Autodesk Fusion 360 part; units mm, degrees
note: some values were not read from the file. Chosen so that the rebuilt part matches the saved one: that a step has no effect.
(part 4 of 7)
  spline S1007 degree 3 poles (-9.5703, 47.6755) (-12.0382, 47.6755) (-14.506, 47.6755) (-17.0486, 47.6755) knots 0 0 0 0 1 1 1 1
  spline S1008 degree 3 poles (-17.0486, 47.6755) (-17.2132, 47.1819) (-17.3777, 46.6884) (-17.5472, 46.1798) knots 0 0 0 0 1 1 1 1
  spline S1009 degree 3 poles (-17.5472, 46.1798) (-17.5472, 46.8379) (-17.5472, 47.496) (-17.5472, 48.1741) knots 0 0 0 0 1 1 1 1
  spline S1010 degree 3 poles (-17.5472, 48.1741) (-16.019, 48.9382) (-14.4225, 48.7239) (-12.7486, 48.7038) knots 0 0 0 0 1 1 1 1
  spline S1011 degree 3 poles (-38.4866, -11.6527) (-38.4866, -12.1462) (-38.4866, -12.6398) (-38.4866, -13.1483) knots 0 0 0 0 1 1 1 1
  spline S1012 degree 3 poles (-38.4866, -13.1483) (-41.777, -13.1483) (-45.0675, -13.1483) (-48.4577, -13.1483) knots 0 0 0 0 1 1 1 1
  spline S1013 degree 3 poles (-48.4577, -13.1483) (-48.4577, -12.8193) (-48.4577, -12.4902) (-48.4577, -12.1512) knots 0 0 0 0 1 1 1 1
  spline S1014 degree 3 poles (-48.4577, -12.1512) (-45.1391, -11.5338) (-41.8532, -11.6071) (-38.4866, -11.6527) knots 0 0 0 0 1 1 1 1
  spline S1015 degree 3 poles (38.2911, 14.2723) (38.1265, 12.9561) (37.962, 11.6399) (37.7925, 10.2838) knots 0 0 0 0 1 1 1 1
  spline S1016 degree 3 poles (37.7925, 10.2838) (37.628, 10.7774) (37.4635, 11.271) (37.294, 11.7795) knots 0 0 0 0 1 1 1 1
  spline S1017 degree 3 poles (37.294, 11.7795) (36.0132, 12.4199) (34.918, 12.4424) (33.4925, 12.5585) knots 0 0 0 0 1 1 1 1
  spline S1018 degree 3 poles (33.4925, 12.5585) (32.9925, 12.6002) (32.4925, 12.642) (31.9773, 12.6851) knots 0 0 0 0 1 1 1 1
  spline S1019 degree 3 poles (31.9773, 12.6851) (31.593, 12.7153) (31.2087, 12.7455) (30.8127, 12.7766) knots 0 0 0 0 1 1 1 1
  spline S1020 degree 3 poles (30.8127, 12.7766) (30.8127, 12.9411) (30.8127, 13.1056) (30.8127, 13.2751) knots 0 0 0 0 1 1 1 1
  spline S1021 degree 3 poles (30.8127, 13.2751) (33.3428, 13.9049) (35.6627, 14.407) (38.2911, 14.2723) knots 0 0 0 0 1 1 1 1
  spline S1022 degree 3 poles (-34.9967, -11.6527) (-34.8321, -11.9817) (-34.6676, -12.3107) (-34.4981, -12.6498) knots 0 0 0 0 1 1 1 1
  spline S1023 degree 3 poles (-34.4981, -12.6498) (-33.84, -12.4852) (-33.1819, -12.3207) (-32.5039, -12.1512) knots 0 0 0 0 1 1 1 1
  spline S1024 degree 3 poles (-32.5039, -12.1512) (-32.5039, -12.3157) (-32.5039, -12.4803) (-32.5039, -12.6498) knots 0 0 0 0 1 1 1 1
  spline S1025 degree 3 poles (-32.5039, -12.6498) (-30.6941, -12.8143) (-28.8844, -12.9788) (-27.0198, -13.1483) knots 0 0 0 0 1 1 1 1
  spline S1026 degree 3 poles (-27.0198, -13.1483) (-26.8552, -12.8193) (-26.6907, -12.4902) (-26.5212, -12.1512) knots 0 0 0 0 1 1 1 1
  spline S1027 degree 3 poles (-26.5212, -12.1512) (-25.4929, -11.8396) (-25.4929, -11.8396) (-24.527, -11.6527) knots 0 0 0 0 1 1 1 1
  spline S1028 degree 3 poles (-24.527, -11.6527) (-24.527, -12.3107) (-24.527, -12.9688) (-24.527, -13.6469) knots 0 0 0 0 1 1 1 1
  spline S1029 degree 3 poles (-24.527, -13.6469) (-27.8175, -13.6469) (-31.1079, -13.6469) (-34.4981, -13.6469) knots 0 0 0 0 1 1 1 1
  spline S1030 degree 3 poles (-34.4981, -13.6469) (-34.6626, -12.9888) (-34.8272, -12.3307) (-34.9967, -11.6527) knots 0 0 0 0 1 1 1 1
  spline S1031 degree 3 poles (-8.0746, 35.2116) (-7.9101, 35.2116) (-7.7456, 35.2116) (-7.5761, 35.2116) knots 0 0 0 0 1 1 1 1
  spline S1032 degree 3 poles (-7.5761, 35.2116) (-7.5761, 34.389) (-7.5761, 33.5664) (-7.5761, 32.7188) knots 0 0 0 0 1 1 1 1
  spline S1033 degree 3 poles (-7.5761, 32.7188) (-6.918, 32.7188) (-6.2599, 32.7188) (-5.5819, 32.7188) knots 0 0 0 0 1 1 1 1
  spline S1034 degree 3 poles (-5.5819, 32.7188) (-5.9109, 31.8962) (-6.24, 31.0736) (-6.579, 30.2261) knots 0 0 0 0 1 1 1 1
  spline S1035 degree 3 poles (-6.579, 30.2261) (-7.2371, 30.7196) (-7.8952, 31.2132) (-8.5732, 31.7217) knots 0 0 0 0 1 1 1 1
  spline S1036 degree 3 poles (-8.5732, 31.7217) (-8.7377, 31.3927) (-8.9022, 31.0636) (-9.0717, 30.7246) knots 0 0 0 0 1 1 1 1
  spline S1037 degree 3 poles (-9.0717, 30.7246) (-10.0589, 30.231) (-10.0589, 30.231) (-11.066, 29.7275) knots 0 0 0 0 1 1 1 1
  spline S1038 degree 3 poles (-11.066, 29.7275) (-10.0788, 31.5373) (-9.0917, 33.347) (-8.0746, 35.2116) knots 0 0 0 0 1 1 1 1
  spline S1039 degree 3 poles (4.8878, -4.6729) (5.6867, -7.0587) (4.9289, -8.9438) (3.8907, -11.1541) knots 0 0 0 0 1 1 1 1
  spline S1040 degree 3 poles (3.8907, -11.1541) (2.8001, -12.1824) (2.8001, -12.1824) (1.8965, -12.6498) knots 0 0 0 0 1 1 1 1
  spline S1041 degree 3 poles (1.8965, -12.6498) (2.7191, -12.8143) (3.5417, -12.9788) (4.3893, -13.1483) knots 0 0 0 0 1 1 1 1
  spline S1042 degree 3 poles (4.3893, -13.1483) (4.3893, -13.3128) (4.3893, -13.4774) (4.3893, -13.6469) knots 0 0 0 0 1 1 1 1
  spline S1043 degree 3 poles (4.3893, -13.6469) (3.2376, -13.6469) (2.0859, -13.6469) (0.8994, -13.6469) knots 0 0 0 0 1 1 1 1
  spline S1044 degree 3 poles (0.8994, -13.6469) (0.8994, -12.9888) (0.8994, -12.3307) (0.8994, -11.6527) knots 0 0 0 0 1 1 1 1
  spline S1045 degree 3 poles (0.8994, -11.6527) (1.2798, -11.2928) (1.6603, -10.9329) (2.0523, -10.5621) knots 0 0 0 0 1 1 1 1
  spline S1046 degree 3 poles (2.0523, -10.5621) (3.7647, -8.77) (4.2569, -7.0271) (4.8878, -4.6729) knots 0 0 0 0 1 1 1 1
  spline S1047 degree 3 poles (-23.0313, 13.7737) (-21.4733, 13.0882) (-21.4733, 13.0882) (-20.5385, 12.278) knots 0 0 0 0 1 1 1 1
  spline S1048 degree 3 poles (-20.5385, 12.278) (-20.5385, 11.949) (-20.5385, 11.6199) (-20.5385, 11.2809) knots 0 0 0 0 1 1 1 1
  spline S1049 degree 3 poles (-20.5385, 11.2809) (-21.0321, 11.1164) (-21.5257, 10.9519) (-22.0342, 10.7824) knots 0 0 0 0 1 1 1 1
  spline S1050 degree 3 poles (-22.0342, 10.7824) (-22.0342, 11.1114) (-22.0342, 11.4405) (-22.0342, 11.7795) knots 0 0 0 0 1 1 1 1
  spline S1051 degree 3 poles (-22.0342, 11.7795) (-22.3633, 11.7795) (-22.6923, 11.7795) (-23.0313, 11.7795) knots 0 0 0 0 1 1 1 1
  spline S1052 degree 3 poles (-23.0313, 11.7795) (-23.0313, 12.1085) (-23.0313, 12.4376) (-23.0313, 12.7766) knots 0 0 0 0 1 1 1 1
  spline S1053 degree 3 poles (-23.0313, 12.7766) (-25.1701, 12.7766) (-27.3089, 12.7766) (-29.5125, 12.7766) knots 0 0 0 0 1 1 1 1
  spline S1054 degree 3 poles (-29.5125, 12.7766) (-27.3952, 14.1881) (-25.5172, 14.0389) (-23.0313, 13.7737) knots 0 0 0 0 1 1 1 1
  spline S1055 degree 3 poles (-67.9014, 21.7506) (-68.5578, 18.9278) (-69.5994, 17.8889) (-71.8898, 16.2665) knots 0 0 0 0 1 1 1 1
  spline S1056 degree 3 poles (-71.8898, 16.2665) (-72.2189, 16.2665) (-72.5479, 16.2665) (-72.8869, 16.2665) knots 0 0 0 0 1 1 1 1
  spline S1057 degree 3 poles (-72.8869, 16.2665) (-72.2127, 17.7316) (-71.4414, 18.905) (-70.3941, 20.1303) knots 0 0 0 0 1 1 1 1
  spline S1058 degree 3 poles (-70.3941, 20.1303) (-70.1371, 20.4362) (-69.88, 20.7421) (-69.6151, 21.0573) knots 0 0 0 0 1 1 1 1
  spline S1059 degree 3 poles (-69.6151, 21.0573) (-68.8985, 21.7506) (-68.8985, 21.7506) (-67.9014, 21.7506) knots 0 0 0 0 1 1 1 1
  spline S1060 degree 3 poles (23.8329, 34.2145) (24.3315, 32.7188) (24.3315, 32.7188) (24.3315, 31.7217) knots 0 0 0 0 1 1 1 1
  spline S1061 degree 3 poles (24.3315, 31.7217) (24.6605, 31.3927) (24.9896, 31.0636) (25.3286, 30.7246) knots 0 0 0 0 1 1 1 1
  spline S1062 degree 3 poles (25.3286, 30.7246) (23.5167, 29.565) (21.9529, 29.6464) (19.8445, 29.7275) knots 0 0 0 0 1 1 1 1
  spline S1063 degree 3 poles (19.8445, 29.7275) (19.68, 30.0565) (19.5155, 30.3856) (19.3459, 30.7246) knots 0 0 0 0 1 1 1 1
  spline S1064 degree 3 poles (19.3459, 30.7246) (20.1686, 30.7246) (20.9912, 30.7246) (21.8387, 30.7246) knots 0 0 0 0 1 1 1 1
  spline S1065 degree 3 poles (21.8387, 30.7246) (21.8387, 31.0537) (21.8387, 31.3827) (21.8387, 31.7217) knots 0 0 0 0 1 1 1 1
  spline S1066 degree 3 poles (21.8387, 31.7217) (22.1678, 31.7217) (22.4968, 31.7217) (22.8358, 31.7217) knots 0 0 0 0 1 1 1 1
  spline S1067 degree 3 poles (22.8358, 31.7217) (22.9078, 32.0405) (22.9798, 32.3592) (23.054, 32.6877) knots 0 0 0 0 1 1 1 1
  spline S1068 degree 3 poles (23.054, 32.6877) (23.3344, 33.7159) (23.3344, 33.7159) (23.8329, 34.2145) knots 0 0 0 0 1 1 1 1
  spline S1069 degree 3 poles (-56.9331, 25.2405) (-54.7943, 25.076) (-52.6555, 24.9114) (-50.4519, 24.7419) knots 0 0 0 0 1 1 1 1
  spline S1070 degree 3 poles (-50.4519, 24.7419) (-50.4519, 23.9193) (-50.4519, 23.0967) (-50.4519, 22.2492) knots 0 0 0 0 1 1 1 1
  spline S1071 degree 3 poles (-50.4519, 22.2492) (-50.727, 22.4073) (-51.002, 22.5653) (-51.2854, 22.7282) knots 0 0 0 0 1 1 1 1
  spline S1072 degree 3 poles (-51.2854, 22.7282) (-52.5881, 23.3096) (-53.6455, 23.4459) (-55.0635, 23.5579) knots 0 0 0 0 1 1 1 1
  spline S1073 degree 3 poles (-55.0635, 23.5579) (-55.5083, 23.5951) (-55.953, 23.6324) (-56.4112, 23.6708) knots 0 0 0 0 1 1 1 1
  spline S1074 degree 3 poles (-56.4112, 23.6708) (-56.9163, 23.7075) (-56.9163, 23.7075) (-57.4317, 23.7448) knots 0 0 0 0 1 1 1 1
  spline S1075 degree 3 poles (-57.4317, 23.7448) (-57.2672, 24.2384) (-57.1026, 24.732) (-56.9331, 25.2405) knots 0 0 0 0 1 1 1 1
  spline S1076 degree 3 poles (-60.9216, -11.6527) (-59.4409, -11.8172) (-57.9602, -11.9817) (-56.4346, -12.1512) knots 0 0 0 0 1 1 1 1
  spline S1077 degree 3 poles (-56.4346, -12.1512) (-58.032, -13.2161) (-58.4268, -13.269) (-60.2575, -13.2457) knots 0 0 0 0 1 1 1 1
  spline S1078 degree 3 poles (-60.2575, -13.2457) (-60.7025, -13.2425) (-61.1476, -13.2393) (-61.6061, -13.236) knots 0 0 0 0 1 1 1 1
  spline S1079 degree 3 poles (-61.6061, -13.236) (-62.3007, -13.2234) (-62.3007, -13.2234) (-63.0093, -13.2106) knots 0 0 0 0 1 1 1 1
  spline S1080 degree 3 poles (-63.0093, -13.2106) (-63.4781, -13.2061) (-63.9469, -13.2016) (-64.43, -13.197) knots 0 0 0 0 1 1 1 1
  spline S1081 degree 3 poles (-64.43, -13.197) (-65.5872, -13.1853) (-66.7442, -13.1689) (-67.9014, -13.1483) knots 0 0 0 0 1 1 1 1
  spline S1082 degree 3 poles (-67.9014, -13.1483) (-67.9014, -12.9838) (-67.9014, -12.8193) (-67.9014, -12.6498) knots 0 0 0 0 1 1 1 1
  spline S1083 degree 3 poles (-67.9014, -12.6498) (-65.598, -12.6498) (-63.2947, -12.6498) (-60.9216, -12.6498) knots 0 0 0 0 1 1 1 1
  spline S1084 degree 3 poles (-60.9216, -12.6498) (-60.9216, -12.3207) (-60.9216, -11.9917) (-60.9216, -11.6527) knots 0 0 0 0 1 1 1 1
  spline S1085 degree 3 poles (-12.5616, -1.6815) (-12.2326, -1.6815) (-11.9035, -1.6815) (-11.5645, -1.6815) knots 0 0 0 0 1 1 1 1
  spline S1086 degree 3 poles (-11.5645, -1.6815) (-11.6352, -2.5542) (-11.7084, -3.4266) (-11.7826, -4.299) knots 0 0 0 0 1 1 1 1
  spline S1087 degree 3 poles (-11.7826, -4.299) (-11.8231, -4.7848) (-11.8636, -5.2707) (-11.9053, -5.7713) knots 0 0 0 0 1 1 1 1
  spline S1088 degree 3 poles (-11.9053, -5.7713) (-12.0385, -6.9486) (-12.2394, -8.0227) (-12.5616, -9.1599) knots 0 0 0 0 1 1 1 1
  spline S1089 degree 3 poles (-12.5616, -9.1599) (-12.5616, -8.8308) (-12.5616, -8.5018) (-12.5616, -8.1628) knots 0 0 0 0 1 1 1 1
  spline S1090 degree 3 poles (-12.5616, -8.1628) (-12.8907, -8.1628) (-13.2197, -8.1628) (-13.5588, -8.1628) knots 0 0 0 0 1 1 1 1
  spline S1091 degree 3 poles (-13.5588, -8.1628) (-14.1196, -5.2961) (-14.1196, -5.2961) (-13.5588, -4.1743) knots 0 0 0 0 1 1 1 1
  spline S1092 degree 3 poles (-13.5588, -4.1743) (-13.2297, -4.1743) (-12.9007, -4.1743) (-12.5616, -4.1743) knots 0 0 0 0 1 1 1 1
  spline S1093 degree 3 poles (-12.5616, -4.1743) (-12.5616, -3.3517) (-12.5616, -2.5291) (-12.5616, -1.6815) knots 0 0 0 0 1 1 1 1
  spline S1094 degree 3 poles (-40.9793, 6.2954) (-40.8148, 6.2954) (-40.6503, 6.2954) (-40.4808, 6.2954) knots 0 0 0 0 1 1 1 1
  spline S1095 degree 3 poles (-40.4808, 6.2954) (-40.402, 2.2758) (-40.402, 2.2758) (-40.9793, 0.3127) knots 0 0 0 0 1 1 1 1
  spline S1096 degree 3 poles (-40.9793, 0.3127) (-41.4729, 0.0659) (-41.4729, 0.0659) (-41.9764, -0.1859) knots 0 0 0 0 1 1 1 1
  spline S1097 degree 3 poles (-41.9764, -0.1859) (-42.5416, -1.1913) (-42.5416, -1.1913) (-42.9736, -2.1801) knots 0 0 0 0 1 1 1 1
  spline S1098 degree 3 poles (-42.9736, -2.1801) (-43.4721, -1.183) (-43.4721, -1.183) (-42.9755, 0.5503) knots 0 0 0 0 1 1 1 1
  spline S1099 degree 3 poles (-42.9755, 0.5503) (-42.7397, 1.241) (-42.5, 1.9304) (-42.2569, 2.6185) knots 0 0 0 0 1 1 1 1
  spline S1100 degree 3 poles (-42.2569, 2.6185) (-42.1357, 2.9707) (-42.0146, 3.3229) (-41.8898, 3.6857) knots 0 0 0 0 1 1 1 1
  spline S1101 degree 3 poles (-41.8898, 3.6857) (-41.5896, 4.5568) (-41.2849, 5.4262) (-40.9793, 6.2954) knots 0 0 0 0 1 1 1 1
  spline S1102 degree 3 poles (41.781, 8.2896) (42.8247, 6.5935) (42.8675, 5.272) (42.7781, 3.304) knots 0 0 0 0 1 1 1 1
  spline S1103 degree 3 poles (42.7781, 3.304) (42.2845, 3.304) (41.7909, 3.304) (41.2824, 3.304) knots 0 0 0 0 1 1 1 1
  spline S1104 degree 3 poles (41.2824, 3.304) (41.2824, 2.4814) (41.2824, 1.6588) (41.2824, 0.8112) knots 0 0 0 0 1 1 1 1
  spline S1105 degree 3 poles (41.2824, 0.8112) (40.9534, 1.1403) (40.6243, 1.4693) (40.2853, 1.8084) knots 0 0 0 0 1 1 1 1
  spline S1106 degree 3 poles (40.2853, 1.8084) (40.4616, 4.1002) (40.9932, 6.1363) (41.781, 8.2896) knots 0 0 0 0 1 1 1 1
  spline S1107 degree 3 poles (-59.9245, 16.765) (-58.4911, 16.8274) (-58.4911, 16.8274) (-56.9331, 16.765) knots 0 0 0 0 1 1 1 1
  spline S1108 degree 3 poles (-56.9331, 16.765) (-55.936, 15.7679) (-55.936, 15.7679) (-55.8737, 14.4592) knots 0 0 0 0 1 1 1 1
  spline S1109 degree 3 poles (-55.8737, 14.4592) (-55.8943, 14.0685) (-55.9148, 13.6777) (-55.936, 13.2751) knots 0 0 0 0 1 1 1 1
  spline S1110 degree 3 poles (-55.936, 13.2751) (-56.4296, 13.2751) (-56.9232, 13.2751) (-57.4317, 13.2751) knots 0 0 0 0 1 1 1 1
  spline S1111 degree 3 poles (-57.4317, 13.2751) (-57.4317, 13.9332) (-57.4317, 14.5913) (-57.4317, 15.2694) knots 0 0 0 0 1 1 1 1
  spline S1112 degree 3 poles (-57.4317, 15.2694) (-58.2543, 15.2694) (-59.0769, 15.2694) (-59.9245, 15.2694) knots 0 0 0 0 1 1 1 1
  spline S1113 degree 3 poles (-59.9245, 15.2694) (-59.9245, 15.7629) (-59.9245, 16.2565) (-59.9245, 16.765) knots 0 0 0 0 1 1 1 1
  spline S1114 degree 3 poles (18.3488, 47.177) (18.3488, 46.8479) (18.3488, 46.5189) (18.3488, 46.1798) knots 0 0 0 0 1 1 1 1
  spline S1115 degree 3 poles (18.3488, 46.1798) (18.0198, 46.1798) (17.6907, 46.1798) (17.3517, 46.1798) knots 0 0 0 0 1 1 1 1
  spline S1116 degree 3 poles (17.3517, 46.1798) (17.2386, 45.8611) (17.1255, 45.5423) (17.009, 45.2139) knots 0 0 0 0 1 1 1 1
  spline S1117 degree 3 poles (17.009, 45.2139) (16.3546, 44.1856) (16.3546, 44.1856) (15.1394, 43.8117) knots 0 0 0 0 1 1 1 1
  spline S1118 degree 3 poles (15.1394, 43.8117) (13.8618, 43.6871) (13.8618, 43.6871) (12.3662, 43.6871) knots 0 0 0 0 1 1 1 1
  spline S1119 degree 3 poles (12.3662, 43.6871) (12.8182, 44.1798) (13.2765, 44.6669) (13.7372, 45.1516) knots 0 0 0 0 1 1 1 1
  spline S1120 degree 3 poles (13.7372, 45.1516) (13.9917, 45.4234) (14.2462, 45.6953) (14.5084, 45.9754) knots 0 0 0 0 1 1 1 1
  spline S1121 degree 3 poles (14.5084, 45.9754) (15.7232, 46.9812) (16.7958, 47.177) (18.3488, 47.177) knots 0 0 0 0 1 1 1 1
  spline S1122 degree 3 poles (-70.3941, 2.8055) (-69.8218, 1.6706) (-69.2707, 0.5346) (-68.7427, -0.6221) knots 0 0 0 0 1 1 1 1
  spline S1123 degree 3 poles (-68.7427, -0.6221) (-67.7966, -2.3741) (-66.7217, -3.6809) (-65.4086, -5.1714) knots 0 0 0 0 1 1 1 1
  spline S1124 degree 3 poles (-65.4086, -5.1714) (-67.3008, -4.3709) (-69.1704, -3.3611) (-70.3941, -1.6815) knots 0 0 0 0 1 1 1 1
  spline S1125 degree 3 poles (-70.3941, -1.6815) (-70.6454, -0.1532) (-70.5746, 1.2717) (-70.3941, 2.8055) knots 0 0 0 0 1 1 1 1
  spline S1126 degree 3 poles (-50.9505, 14.7708) (-49.9533, 13.7737) (-49.9533, 13.7737) (-49.9533, 12.278) knots 0 0 0 0 1 1 1 1
  spline S1127 degree 3 poles (-49.9533, 12.278) (-50.2824, 12.278) (-50.6114, 12.278) (-50.9505, 12.278) knots 0 0 0 0 1 1 1 1
  spline S1128 degree 3 poles (-50.9505, 12.278) (-50.9505, 11.949) (-50.9505, 11.6199) (-50.9505, 11.2809) knots 0 0 0 0 1 1 1 1
  spline S1129 degree 3 poles (-50.9505, 11.2809) (-51.2795, 11.2809) (-51.6085, 11.2809) (-51.9476, 11.2809) knots 0 0 0 0 1 1 1 1
  spline S1130 degree 3 poles (-51.9476, 11.2809) (-52.1121, 10.7874) (-52.2766, 10.2938) (-52.4461, 9.7853) knots 0 0 0 0 1 1 1 1
  spline S1131 degree 3 poles (-52.4461, 9.7853) (-53.2687, 9.7853) (-54.0914, 9.7853) (-54.9389, 9.7853) knots 0 0 0 0 1 1 1 1
  spline S1132 degree 3 poles (-54.9389, 9.7853) (-54.7345, 10.0198) (-54.5302, 10.2544) (-54.3196, 10.4961) knots 0 0 0 0 1 1 1 1
  spline S1133 degree 3 poles (-54.3196, 10.4961) (-54.051, 10.8065) (-53.7823, 11.1169) (-53.5056, 11.4367) knots 0 0 0 0 1 1 1 1
  spline S1134 degree 3 poles (-53.5056, 11.4367) (-53.2395, 11.7433) (-52.9734, 12.0498) (-52.6993, 12.3657) knots 0 0 0 0 1 1 1 1
  spline S1135 degree 3 poles (-52.6993, 12.3657) (-51.8658, 13.3424) (-51.8658, 13.3424) (-50.9505, 14.7708) knots 0 0 0 0 1 1 1 1
  spline S1136 degree 3 poles (-8.5732, 31.7217) (-8.0796, 31.5572) (-7.5861, 31.3927) (-7.0775, 31.2232) knots 0 0 0 0 1 1 1 1
  spline S1137 degree 3 poles (-7.0775, 31.2232) (-7.0152, 30.0391) (-7.0152, 30.0391) (-7.0775, 28.7304) knots 0 0 0 0 1 1 1 1
  spline S1138 degree 3 poles (-7.0775, 28.7304) (-7.4066, 28.4013) (-7.7356, 28.0723) (-8.0746, 27.7333) knots 0 0 0 0 1 1 1 1
  spline S1139 degree 3 poles (-8.0746, 27.7333) (-8.7327, 27.7333) (-9.3908, 27.7333) (-10.0689, 27.7333) knots 0 0 0 0 1 1 1 1
  spline S1140 degree 3 poles (-10.0689, 27.7333) (-9.756, 29.1934) (-9.278, 30.406) (-8.5732, 31.7217) knots 0 0 0 0 1 1 1 1
  spline S1141 degree 3 poles (5.8849, -1.6815) (7.0746, -3.466) (7.1206, -4.0613) (6.882, -6.1685) knots 0 0 0 0 1 1 1 1
  spline S1142 degree 3 poles (6.882, -6.1685) (6.3086, -7.5522) (5.6277, -8.8556) (4.8878, -10.157) knots 0 0 0 0 1 1 1 1
  spline S1143 degree 3 poles (4.8878, -10.157) (4.0942, -8.5697) (4.7445, -7.0257) (5.1059, -5.3584) knots 0 0 0 0 1 1 1 1
  spline S1144 degree 3 poles (5.1059, -5.3584) (5.1795, -5.0062) (5.2531, -4.654) (5.3289, -4.2912) knots 0 0 0 0 1 1 1 1
  spline S1145 degree 3 poles (5.3289, -4.2912) (5.5113, -3.4207) (5.6977, -2.551) (5.8849, -1.6815) knots 0 0 0 0 1 1 1 1
  spline S1146 degree 3 poles (-9.5703, 14.2723) (-8.5832, 14.2723) (-7.596, 14.2723) (-6.579, 14.2723) knots 0 0 0 0 1 1 1 1
  spline S1147 degree 3 poles (-6.579, 14.2723) (-6.818, 11.922) (-7.0617, 9.9519) (-8.0746, 7.791) knots 0 0 0 0 1 1 1 1
  spline S1148 degree 3 poles (-8.0746, 7.791) (-8.4172, 9.0328) (-8.5732, 9.9741) (-8.5732, 11.2809) knots 0 0 0 0 1 1 1 1
  spline S1149 degree 3 poles (-8.5732, 11.2809) (-8.7377, 11.4454) (-8.9022, 11.61) (-9.0717, 11.7795) knots 0 0 0 0 1 1 1 1
  spline S1150 degree 3 poles (-9.0717, 11.7795) (-9.0717, 12.1085) (-9.0717, 12.4376) (-9.0717, 12.7766) knots 0 0 0 0 1 1 1 1
  spline S1151 degree 3 poles (-9.0717, 12.7766) (-8.7427, 12.7766) (-8.4137, 12.7766) (-8.0746, 12.7766) knots 0 0 0 0 1 1 1 1
  spline S1152 degree 3 poles (-8.0746, 12.7766) (-8.0746, 13.1056) (-8.0746, 13.4347) (-8.0746, 13.7737) knots 0 0 0 0 1 1 1 1
  spline S1153 degree 3 poles (-8.0746, 13.7737) (-8.5682, 13.9382) (-9.0618, 14.1028) (-9.5703, 14.2723) knots 0 0 0 0 1 1 1 1
  spline S1154 degree 3 poles (-61.4201, 23.7448) (-61.0911, 23.2513) (-60.762, 22.7577) (-60.423, 22.2492) knots 0 0 0 0 1 1 1 1
  spline S1155 degree 3 poles (-60.423, 22.2492) (-61.1492, 21.6768) (-61.8765, 21.1058) (-62.6042, 20.5354) knots 0 0 0 0 1 1 1 1
  spline S1156 degree 3 poles (-62.6042, 20.5354) (-63.0091, 20.2172) (-63.414, 19.8991) (-63.8311, 19.5714) knots 0 0 0 0 1 1 1 1
  spline S1157 degree 3 poles (-63.8311, 19.5714) (-64.91, 18.7593) (-64.91, 18.7593) (-65.9071, 18.2607) knots 0 0 0 0 1 1 1 1
  spline S1158 degree 3 poles (-65.9071, 18.2607) (-65.7513, 19.2267) (-65.7513, 19.2267) (-65.4086, 20.2549) knots 0 0 0 0 1 1 1 1
  spline S1159 degree 3 poles (-65.4086, 20.2549) (-64.915, 20.4195) (-64.4214, 20.584) (-63.9129, 20.7535) knots 0 0 0 0 1 1 1 1
  spline S1160 degree 3 poles (-63.9129, 20.7535) (-63.572, 21.4139) (-63.24, 22.079) (-62.9158, 22.7477) knots 0 0 0 0 1 1 1 1
  spline S1161 degree 3 poles (-62.9158, 22.7477) (-62.4222, 23.0768) (-61.9287, 23.4058) (-61.4201, 23.7448) knots 0 0 0 0 1 1 1 1
  spline S1162 degree 3 poles (26.3257, 6.2954) (26.8193, 6.1308) (27.3129, 5.9663) (27.8214, 5.7968) knots 0 0 0 0 1 1 1 1
  spline S1163 degree 3 poles (27.8214, 5.7968) (27.2917, 4.6127) (27.2917, 4.6127) (26.3257, 3.304) knots 0 0 0 0 1 1 1 1
  spline S1164 degree 3 poles (26.3257, 3.304) (24.4873, 2.6497) (24.4873, 2.6497) (22.8358, 2.3069) knots 0 0 0 0 1 1 1 1
  spline S1165 degree 3 poles (22.8358, 2.3069) (22.5068, 2.636) (22.1777, 2.965) (21.8387, 3.304) knots 0 0 0 0 1 1 1 1
  spline S1166 degree 3 poles (21.8387, 3.304) (22.6613, 3.304) (23.484, 3.304) (24.3315, 3.304) knots 0 0 0 0 1 1 1 1
  spline S1167 degree 3 poles (24.3315, 3.304) (24.4086, 3.7667) (24.4086, 3.7667) (24.4873, 4.2388) knots 0 0 0 0 1 1 1 1
  spline S1168 degree 3 poles (24.4873, 4.2388) (24.8301, 5.2983) (24.8301, 5.2983) (26.3257, 6.2954) knots 0 0 0 0 1 1 1 1
  spline S1169 degree 3 poles (-36.9909, 19.2578) (-36.8264, 19.2578) (-36.6618, 19.2578) (-36.4923, 19.2578) knots 0 0 0 0 1 1 1 1
  spline S1170 degree 3 poles (-36.4923, 19.2578) (-36.2215, 15.9397) (-36.6055, 14.0437) (-38.4866, 11.2809) knots 0 0 0 0 1 1 1 1
  spline S1171 degree 3 poles (-38.4866, 11.2809) (-39.1408, 13.2436) (-38.6558, 14.1623) (-38.0192, 16.1107) knots 0 0 0 0 1 1 1 1
  spline S1172 degree 3 poles (-38.0192, 16.1107) (-37.8296, 16.6987) (-37.64, 17.2868) (-37.4446, 17.8926) knots 0 0 0 0 1 1 1 1
  spline S1173 degree 3 poles (-37.4446, 17.8926) (-37.2949, 18.3431) (-37.1452, 18.7937) (-36.9909, 19.2578) knots 0 0 0 0 1 1 1 1
  spline S1174 degree 3 poles (5.0787, 48.77) (5.5298, 48.7584) (5.981, 48.7469) (6.4458, 48.7349) knots 0 0 0 0 1 1 1 1
  spline S1175 degree 3 poles (6.4458, 48.7349) (7.1264, 48.7214) (7.1264, 48.7214) (7.8207, 48.7077) knots 0 0 0 0 1 1 1 1
  spline S1176 degree 3 poles (7.8207, 48.7077) (8.1691, 48.6961) (8.5174, 48.6845) (8.8763, 48.6726) knots 0 0 0 0 1 1 1 1
  spline S1177 degree 3 poles (8.8763, 48.6726) (9.256, 46.5206) (9.4549, 44.8116) (8.8763, 42.69) knots 0 0 0 0 1 1 1 1
  spline S1178 degree 3 poles (8.8763, 42.69) (8.7117, 42.69) (8.5472, 42.69) (8.3777, 42.69) knots 0 0 0 0 1 1 1 1
  spline S1179 degree 3 poles (8.3777, 42.69) (8.2132, 44.3352) (8.0487, 45.9804) (7.8792, 47.6755) knots 0 0 0 0 1 1 1 1
  spline S1180 degree 3 poles (7.8792, 47.6755) (6.2339, 47.6755) (4.5887, 47.6755) (2.8936, 47.6755) knots 0 0 0 0 1 1 1 1
  spline S1181 degree 3 poles (2.8936, 47.6755) (3.8907, 48.6726) (3.8907, 48.6726) (5.0787, 48.77) knots 0 0 0 0 1 1 1 1
  spline S1182 degree 3 poles (36.2968, 7.2925) (36.1548, 6.5855) (36.0086, 5.8794) (35.8606, 5.1736) knots 0 0 0 0 1 1 1 1
  spline S1183 degree 3 poles (35.8606, 5.1736) (35.7391, 4.5836) (35.7391, 4.5836) (35.6152, 3.9818) knots 0 0 0 0 1 1 1 1
  spline S1184 degree 3 poles (35.6152, 3.9818) (35.304, 2.8213) (34.8768, 1.863) (34.3026, 0.8112) knots 0 0 0 0 1 1 1 1
  spline S1185 degree 3 poles (34.3026, 0.8112) (34.1783, 1.6095) (34.0664, 2.4097) (33.9599, 3.2105) knots 0 0 0 0 1 1 1 1
  spline S1186 degree 3 poles (33.9599, 3.2105) (33.8962, 3.6559) (33.8326, 4.1013) (33.7671, 4.5602) knots 0 0 0 0 1 1 1 1
  spline S1187 degree 3 poles (33.7671, 4.5602) (33.8041, 5.7968) (33.8041, 5.7968) (34.4798, 6.7063) knots 0 0 0 0 1 1 1 1
  spline S1188 degree 3 poles (34.4798, 6.7063) (35.2997, 7.2925) (35.2997, 7.2925) (36.2968, 7.2925) knots 0 0 0 0 1 1 1 1
  spline S1189 degree 3 poles (-61.9187, 6.7939) (-61.2606, 6.7939) (-60.6025, 6.7939) (-59.9245, 6.7939) knots 0 0 0 0 1 1 1 1
  spline S1190 degree 3 poles (-59.9245, 6.7939) (-59.9245, 6.4649) (-59.9245, 6.1358) (-59.9245, 5.7968) knots 0 0 0 0 1 1 1 1
  spline S1191 degree 3 poles (-59.9245, 5.7968) (-58.9373, 5.9613) (-57.9502, 6.1259) (-56.9331, 6.2954) knots 0 0 0 0 1 1 1 1
  spline S1192 degree 3 poles (-56.9331, 6.2954) (-56.7686, 5.9663) (-56.6041, 5.6373) (-56.4346, 5.2983) knots 0 0 0 0 1 1 1 1
  spline S1193 degree 3 poles (-56.4346, 5.2983) (-54.9243, 4.9703) (-54.9243, 4.9703) (-53.4432, 4.7997) knots 0 0 0 0 1 1 1 1
  spline S1194 degree 3 poles (-53.4432, 4.7997) (-53.4432, 4.6352) (-53.4432, 4.4706) (-53.4432, 4.3011) knots 0 0 0 0 1 1 1 1
  spline S1195 degree 3 poles (-53.4432, 4.3011) (-56.529, 4.1358) (-58.5981, 4.5096) (-61.4201, 5.7968) knots 0 0 0 0 1 1 1 1
  spline S1196 degree 3 poles (-61.4201, 5.7968) (-61.5847, 6.1259) (-61.7492, 6.4549) (-61.9187, 6.7939) knots 0 0 0 0 1 1 1 1
  spline S1197 degree 3 poles (-12.5616, 32.2203) (-12.2326, 31.8912) (-11.9035, 31.5622) (-11.5645, 31.2232) knots 0 0 0 0 1 1 1 1
  spline S1198 degree 3 poles (-11.5645, 31.2232) (-11.7291, 30.5651) (-11.8936, 29.907) (-12.0631, 29.2289) knots 0 0 0 0 1 1 1 1
  spline S1199 degree 3 poles (-12.0631, 29.2289) (-14.6955, 29.2289) (-17.3278, 29.2289) (-20.04, 29.2289) knots 0 0 0 0 1 1 1 1
  spline S1200 degree 3 poles (-20.04, 29.2289) (-20.04, 29.3935) (-20.04, 29.558) (-20.04, 29.7275) knots 0 0 0 0 1 1 1 1
  spline S1201 degree 3 poles (-20.04, 29.7275) (-18.0657, 29.7275) (-16.0914, 29.7275) (-14.0573, 29.7275) knots 0 0 0 0 1 1 1 1
  spline S1202 degree 3 poles (-14.0573, 29.7275) (-14.0573, 30.0565) (-14.0573, 30.3856) (-14.0573, 30.7246) knots 0 0 0 0 1 1 1 1
  spline S1203 degree 3 poles (-14.0573, 30.7246) (-13.5637, 30.7246) (-13.0702, 30.7246) (-12.5616, 30.7246) knots 0 0 0 0 1 1 1 1
  spline S1204 degree 3 poles (-12.5616, 30.7246) (-12.5616, 31.2182) (-12.5616, 31.7117) (-12.5616, 32.2203) knots 0 0 0 0 1 1 1 1
  spline S1205 degree 3 poles (20.8416, 47.6755) (22.9804, 47.6755) (25.1192, 47.6755) (27.3228, 47.6755) knots 0 0 0 0 1 1 1 1
  spline S1206 degree 3 poles (27.3228, 47.6755) (27.3228, 47.3465) (27.3228, 47.0174) (27.3228, 46.6784) knots 0 0 0 0 1 1 1 1
  spline S1207 degree 3 poles (27.3228, 46.6784) (26.8447, 46.6013) (26.8447, 46.6013) (26.3569, 46.5226) knots 0 0 0 0 1 1 1 1
  spline S1208 degree 3 poles (26.3569, 46.5226) (26.0176, 46.4095) (25.6782, 46.2964) (25.3286, 46.1798) knots 0 0 0 0 1 1 1 1
  spline S1209 degree 3 poles (25.3286, 46.1798) (25.1641, 45.6863) (24.9996, 45.1927) (24.8301, 44.6842) knots 0 0 0 0 1 1 1 1
  spline S1210 degree 3 poles (24.8301, 44.6842) (24.501, 45.1777) (24.172, 45.6713) (23.8329, 46.1798) knots 0 0 0 0 1 1 1 1
  spline S1211 degree 3 poles (23.8329, 46.1798) (22.3102, 46.7845) (22.3102, 46.7845) (20.8416, 47.177) knots 0 0 0 0 1 1 1 1
  spline S1212 degree 3 poles (20.8416, 47.177) (20.8416, 47.3415) (20.8416, 47.506) (20.8416, 47.6755) knots 0 0 0 0 1 1 1 1
  spline S1213 degree 3 poles (2.395, 4.7997) (2.7241, 4.7997) (3.0531, 4.7997) (3.3922, 4.7997) knots 0 0 0 0 1 1 1 1
  spline S1214 degree 3 poles (3.3922, 4.7997) (3.2508, 4.0822) (3.1044, 3.3657) (2.9559, 2.6497) knots 0 0 0 0 1 1 1 1
  spline S1215 degree 3 poles (2.9559, 2.6497) (2.8749, 2.2506) (2.794, 1.8515) (2.7105, 1.4403) knots 0 0 0 0 1 1 1 1
  spline S1216 degree 3 poles (2.7105, 1.4403) (2.395, 0.3127) (2.395, 0.3127) (1.3979, -1.183) knots 0 0 0 0 1 1 1 1
  spline S1217 degree 3 poles (1.3979, -1.183) (0.3385, 1.1228) (0.3385, 1.1228) (0.8994, 2.8055) knots 0 0 0 0 1 1 1 1
  spline S1218 degree 3 poles (0.8994, 2.8055) (1.2284, 2.97) (1.5575, 3.1345) (1.8965, 3.304) knots 0 0 0 0 1 1 1 1
  spline S1219 degree 3 poles (1.8965, 3.304) (2.061, 3.7976) (2.2255, 4.2912) (2.395, 4.7997) knots 0 0 0 0 1 1 1 1
  spline S1220 degree 3 poles (23.3344, 10.2838) (23.7083, 9.4113) (23.7083, 9.4113) (23.8329, 8.2896) knots 0 0 0 0 1 1 1 1
  spline S1221 degree 3 poles (23.8329, 8.2896) (23.1682, 7.6248) (22.5035, 6.9601) (21.8387, 6.2954) knots 0 0 0 0 1 1 1 1
  spline S1222 degree 3 poles (21.8387, 6.2954) (21.4383, 4.7275) (21.4383, 4.7275) (21.3402, 3.304) knots 0 0 0 0 1 1 1 1
  spline S1223 degree 3 poles (21.3402, 3.304) (20.3431, 4.3011) (20.3431, 4.3011) (20.1561, 5.4852) knots 0 0 0 0 1 1 1 1
  spline S1224 degree 3 poles (20.1561, 5.4852) (20.399, 7.1852) (21.0133, 7.7368) (22.3373, 8.7881) knots 0 0 0 0 1 1 1 1
  spline S1225 degree 3 poles (22.3373, 8.7881) (22.6663, 8.7881) (22.9954, 8.7881) (23.3344, 8.7881) knots 0 0 0 0 1 1 1 1
  spline S1226 degree 3 poles (23.3344, 8.7881) (23.3344, 9.2817) (23.3344, 9.7753) (23.3344, 10.2838) knots 0 0 0 0 1 1 1 1
  spline S1227 degree 3 poles (5.8849, 13.2751) (5.5559, 12.6171) (5.2268, 11.959) (4.8878, 11.2809) knots 0 0 0 0 1 1 1 1
  spline S1228 degree 3 poles (4.8878, 11.2809) (4.7233, 11.61) (4.5588, 11.939) (4.3893, 12.278) knots 0 0 0 0 1 1 1 1
  spline S1229 degree 3 poles (4.3893, 12.278) (3.3294, 12.5106) (3.3294, 12.5106) (2.1146, 12.5896) knots 0 0 0 0 1 1 1 1
  spline S1230 degree 3 poles (2.1146, 12.5896) (1.7026, 12.6269) (1.2907, 12.6642) (0.8663, 12.7026) knots 0 0 0 0 1 1 1 1
  spline S1231 degree 3 poles (0.8663, 12.7026) (0.5481, 12.727) (0.23, 12.7514) (-0.0977, 12.7766) knots 0 0 0 0 1 1 1 1
  spline S1232 degree 3 poles (-0.0977, 12.7766) (-0.0977, 12.4475) (-0.0977, 12.1185) (-0.0977, 11.7795) knots 0 0 0 0 1 1 1 1
  spline S1233 degree 3 poles (-0.0977, 11.7795) (-0.7558, 11.944) (-1.4139, 12.1085) (-2.092, 12.278) knots 0 0 0 0 1 1 1 1
  spline S1234 degree 3 poles (-2.092, 12.278) (-0.6195, 13.2597) (-0.0689, 13.4446) (1.616, 13.6179) knots 0 0 0 0 1 1 1 1
  spline S1235 degree 3 poles (1.616, 13.6179) (2.1858, 13.6825) (2.1858, 13.6825) (2.767, 13.7484) knots 0 0 0 0 1 1 1 1
  spline S1236 degree 3 poles (2.767, 13.7484) (3.9067, 13.7741) (4.7986, 13.6043) (5.8849, 13.2751) knots 0 0 0 0 1 1 1 1
  spline S1237 degree 3 poles (-47.4606, -4.1743) (-47.6251, -4.6679) (-47.7896, -5.1615) (-47.9591, -5.67) knots 0 0 0 0 1 1 1 1
  spline S1238 degree 3 poles (-47.9591, -5.67) (-48.4527, -5.5055) (-48.9463, -5.3409) (-49.4548, -5.1714) knots 0 0 0 0 1 1 1 1
  spline S1239 degree 3 poles (-49.4548, -5.1714) (-49.4548, -5.8295) (-49.4548, -6.4876) (-49.4548, -7.1656) knots 0 0 0 0 1 1 1 1
  spline S1240 degree 3 poles (-49.4548, -7.1656) (-49.9484, -7.1656) (-50.4419, -7.1656) (-50.9505, -7.1656) knots 0 0 0 0 1 1 1 1
  spline S1241 degree 3 poles (-50.9505, -7.1656) (-50.9505, -6.1785) (-50.9505, -5.1914) (-50.9505, -4.1743) knots 0 0 0 0 1 1 1 1
  spline S1242 degree 3 poles (-50.9505, -4.1743) (-48.5823, -3.6134) (-48.5823, -3.6134) (-47.4606, -4.1743) knots 0 0 0 0 1 1 1 1
  spline S1243 degree 3 poles (39.7867, 1.8084) (39.9513, 1.3148) (40.1158, 0.8212) (40.2853, 0.3127) knots 0 0 0 0 1 1 1 1
  spline S1244 degree 3 poles (40.2853, 0.3127) (40.7789, 0.4772) (41.2724, 0.6417) (41.781, 0.8112) knots 0 0 0 0 1 1 1 1
  spline S1245 degree 3 poles (41.781, 0.8112) (41.4519, -0.0114) (41.1229, -0.834) (40.7839, -1.6815) knots 0 0 0 0 1 1 1 1
  spline S1246 degree 3 poles (40.7839, -1.6815) (40.2903, -1.6815) (39.7967, -1.6815) (39.2882, -1.6815) knots 0 0 0 0 1 1 1 1
  spline S1247 degree 3 poles (39.2882, -1.6815) (39.1237, -2.5042) (38.9591, -3.3268) (38.7896, -4.1743) knots 0 0 0 0 1 1 1 1
  spline S1248 degree 3 poles (38.7896, -4.1743) (38.2294, -2.5269) (38.3431, -1.6563) (39.0077, -0.0612) knots 0 0 0 0 1 1 1 1
  spline S1249 degree 3 poles (39.0077, -0.0612) (39.1511, 0.291) (39.2944, 0.6431) (39.442, 1.006) knots 0 0 0 0 1 1 1 1
  spline S1250 degree 3 poles (39.442, 1.006) (39.5558, 1.2708) (39.6695, 1.5356) (39.7867, 1.8084) knots 0 0 0 0 1 1 1 1
  spline S1251 degree 3 poles (47.7636, 4.3011) (48.3417, 2.5668) (48.1498, 2.1363) (47.5455, 0.4685) knots 0 0 0 0 1 1 1 1
  spline S1252 degree 3 poles (47.5455, 0.4685) (47.4022, 0.0655) (47.2589, -0.3374) (47.1112, -0.7526) knots 0 0 0 0 1 1 1 1
  spline S1253 degree 3 poles (47.1112, -0.7526) (46.9975, -1.0591) (46.8837, -1.3657) (46.7665, -1.6815) knots 0 0 0 0 1 1 1 1
  spline S1254 degree 3 poles (46.7665, -1.6815) (46.602, -1.188) (46.4375, -0.6944) (46.268, -0.1859) knots 0 0 0 0 1 1 1 1
  spline S1255 degree 3 poles (46.268, -0.1859) (45.9389, -0.0213) (45.6099, 0.1432) (45.2709, 0.3127) knots 0 0 0 0 1 1 1 1
  spline S1256 degree 3 poles (45.2709, 0.3127) (45.1063, 0.6417) (44.9418, 0.9708) (44.7723, 1.3098) knots 0 0 0 0 1 1 1 1
  spline S1257 degree 3 poles (44.7723, 1.3098) (45.1013, 1.3098) (45.4304, 1.3098) (45.7694, 1.3098) knots 0 0 0 0 1 1 1 1
  spline S1258 degree 3 poles (45.7694, 1.3098) (45.7694, 1.6389) (45.7694, 1.9679) (45.7694, 2.3069) knots 0 0 0 0 1 1 1 1
  spline S1259 degree 3 poles (45.7694, 2.3069) (46.263, 2.3069) (46.7566, 2.3069) (47.2651, 2.3069) knots 0 0 0 0 1 1 1 1
  spline S1260 degree 3 poles (47.2651, 2.3069) (47.4296, 2.965) (47.5941, 3.6231) (47.7636, 4.3011) knots 0 0 0 0 1 1 1 1
  spline S1261 degree 3 poles (25.3286, -2.6786) (25.8222, -2.8432) (26.3158, -3.0077) (26.8243, -3.1772) knots 0 0 0 0 1 1 1 1
  spline S1262 degree 3 poles (26.8243, -3.1772) (26.8243, -3.8353) (26.8243, -4.4934) (26.8243, -5.1714) knots 0 0 0 0 1 1 1 1
  spline S1263 degree 3 poles (26.8243, -5.1714) (26.4952, -5.1714) (26.1662, -5.1714) (25.8272, -5.1714) knots 0 0 0 0 1 1 1 1
  spline S1264 degree 3 poles (25.8272, -5.1714) (25.8272, -5.994) (25.8272, -6.8167) (25.8272, -7.6642) knots 0 0 0 0 1 1 1 1
  spline S1265 degree 3 poles (25.8272, -7.6642) (25.3336, -7.6642) (24.84, -7.6642) (24.3315, -7.6642) knots 0 0 0 0 1 1 1 1
  spline S1266 degree 3 poles (24.3315, -7.6642) (24.6605, -6.019) (24.9896, -4.3737) (25.3286, -2.6786) knots 0 0 0 0 1 1 1 1
  spline S1267 degree 3 poles (-60.423, 11.7795) (-59.2714, 11.7795) (-58.1197, 11.7795) (-56.9331, 11.7795) knots 0 0 0 0 1 1 1 1
  spline S1268 degree 3 poles (-56.9331, 11.7795) (-56.9331, 11.615) (-56.9331, 11.4504) (-56.9331, 11.2809) knots 0 0 0 0 1 1 1 1
  spline S1269 degree 3 poles (-56.9331, 11.2809) (-57.7557, 11.1164) (-58.5784, 10.9519) (-59.4259, 10.7824) knots 0 0 0 0 1 1 1 1
  spline S1270 degree 3 poles (-59.4259, 10.7824) (-59.2614, 10.4533) (-59.0969, 10.1243) (-58.9274, 9.7853) knots 0 0 0 0 1 1 1 1
  spline S1271 degree 3 poles (-58.9274, 9.7853) (-57.6112, 9.7853) (-56.295, 9.7853) (-54.9389, 9.7853) knots 0 0 0 0 1 1 1 1
  spline S1272 degree 3 poles (-54.9389, 9.7853) (-54.9389, 9.4562) (-54.9389, 9.1272) (-54.9389, 8.7881) knots 0 0 0 0 1 1 1 1
  spline S1273 degree 3 poles (-54.9389, 8.7881) (-55.6554, 8.7611) (-56.3721, 8.7418) (-57.0889, 8.7258) knots 0 0 0 0 1 1 1 1
  spline S1274 degree 3 poles (-57.0889, 8.7258) (-57.488, 8.7143) (-57.8871, 8.7027) (-58.2983, 8.6908) knots 0 0 0 0 1 1 1 1
  spline S1275 degree 3 poles (-58.2983, 8.6908) (-59.4259, 8.7881) (-59.4259, 8.7881) (-60.9216, 9.7853) knots 0 0 0 0 1 1 1 1
  spline S1276 degree 3 poles (-60.9216, 9.7853) (-60.7571, 10.4433) (-60.5925, 11.1014) (-60.423, 11.7795) knots 0 0 0 0 1 1 1 1
  spline S1277 degree 3 poles (-36.9909, -2.6786) (-36.2884, -4.0836) (-36.7373, -4.759) (-37.209, -6.2309) knots 0 0 0 0 1 1 1 1
  spline S1278 degree 3 poles (-37.209, -6.2309) (-37.3523, -6.6846) (-37.4956, -7.1383) (-37.6433, -7.6058) knots 0 0 0 0 1 1 1 1
  spline S1279 degree 3 poles (-37.6433, -7.6058) (-37.757, -7.9541) (-37.8708, -8.3024) (-37.988, -8.6613) knots 0 0 0 0 1 1 1 1
  spline S1280 degree 3 poles (-37.988, -8.6613) (-38.4816, -8.4968) (-38.9751, -8.3323) (-39.4837, -8.1628) knots 0 0 0 0 1 1 1 1
  spline S1281 degree 3 poles (-39.4837, -8.1628) (-39.0474, -5.7946) (-39.0474, -5.7946) (-38.4866, -4.6729) knots 0 0 0 0 1 1 1 1
  spline S1282 degree 3 poles (-38.4866, -4.6729) (-38.1575, -4.6729) (-37.8285, -4.6729) (-37.4894, -4.6729) knots 0 0 0 0 1 1 1 1
  spline S1283 degree 3 poles (-37.4894, -4.6729) (-37.3249, -4.0148) (-37.1604, -3.3567) (-36.9909, -2.6786) knots 0 0 0 0 1 1 1 1
  spline S1284 degree 3 poles (-25.0255, -2.1801) (-24.532, -2.3446) (-24.0384, -2.5091) (-23.5299, -2.6786) knots 0 0 0 0 1 1 1 1
  spline S1285 degree 3 poles (-23.5299, -2.6786) (-24.2702, -5.3933) (-24.2702, -5.3933) (-25.0255, -8.1628) knots 0 0 0 0 1 1 1 1
  spline S1286 degree 3 poles (-25.0255, -8.1628) (-25.1901, -8.1628) (-25.3546, -8.1628) (-25.5241, -8.1628) knots 0 0 0 0 1 1 1 1
  spline S1287 degree 3 poles (-25.5241, -8.1628) (-25.6351, -7.4472) (-25.7373, -6.7302) (-25.8357, -6.0127) knots 0 0 0 0 1 1 1 1
  spline S1288 degree 3 poles (-25.8357, -6.0127) (-25.8935, -5.6136) (-25.9514, -5.2145) (-26.011, -4.8034) knots 0 0 0 0 1 1 1 1
  spline S1289 degree 3 poles (-26.011, -4.8034) (-26.0227, -3.6758) (-26.0227, -3.6758) (-25.0255, -2.1801) knots 0 0 0 0 1 1 1 1
  spline S1290 degree 3 poles (-62.9158, 13.7737) (-61.8647, 12.0657) (-61.8757, 10.7638) (-61.9187, 8.7881) knots 0 0 0 0 1 1 1 1
  spline S1291 degree 3 poles (-61.9187, 8.7881) (-61.7542, 8.4591) (-61.5896, 8.13) (-61.4201, 7.791) knots 0 0 0 0 1 1 1 1
  spline S1292 degree 3 poles (-61.4201, 7.791) (-61.7492, 7.462) (-62.0782, 7.1329) (-62.4172, 6.7939) knots 0 0 0 0 1 1 1 1
  spline S1293 degree 3 poles (-62.4172, 6.7939) (-63.5799, 8.6106) (-63.5298, 10.1608) (-63.4144, 12.278) knots 0 0 0 0 1 1 1 1
  spline S1294 degree 3 poles (-63.4144, 12.278) (-63.2498, 12.7716) (-63.0853, 13.2652) (-62.9158, 13.7737) knots 0 0 0 0 1 1 1 1
  spline S1295 degree 3 poles (-26.0227, 48.1741) (-25.6936, 47.845) (-25.3646, 47.516) (-25.0255, 47.177) knots 0 0 0 0 1 1 1 1
  spline S1296 degree 3 poles (-25.0255, 47.177) (-25.9703, 46.2322) (-27.3046, 46.5886) (-28.5602, 46.5635) knots 0 0 0 0 1 1 1 1
  spline S1297 degree 3 poles (-28.5602, 46.5635) (-29.5125, 46.6784) (-29.5125, 46.6784) (-30.5097, 47.6755) knots 0 0 0 0 1 1 1 1
  spline S1298 degree 3 poles (-30.5097, 47.6755) (-29.0074, 48.4266) (-27.6764, 48.2627) (-26.0227, 48.1741) knots 0 0 0 0 1 1 1 1
  spline S1299 degree 3 poles (13.3633, 11.7795) (13.8568, 11.615) (14.3504, 11.4504) (14.8589, 11.2809) knots 0 0 0 0 1 1 1 1
  spline S1300 degree 3 poles (14.8589, 11.2809) (14.8589, 10.9519) (14.8589, 10.6228) (14.8589, 10.2838) knots 0 0 0 0 1 1 1 1
  spline S1301 degree 3 poles (14.8589, 10.2838) (15.517, 9.9548) (16.1751, 9.6257) (16.8532, 9.2867) knots 0 0 0 0 1 1 1 1
  spline S1302 degree 3 poles (16.8532, 9.2867) (16.6886, 8.9577) (16.5241, 8.6286) (16.3546, 8.2896) knots 0 0 0 0 1 1 1 1
  spline S1303 degree 3 poles (16.3546, 8.2896) (14.8901, 8.6947) (14.8901, 8.6947) (13.3633, 9.2867) knots 0 0 0 0 1 1 1 1
  spline S1304 degree 3 poles (13.3633, 9.2867) (13.1987, 9.7803) (13.0342, 10.2738) (12.8647, 10.7824) knots 0 0 0 0 1 1 1 1
  spline S1305 degree 3 poles (12.8647, 10.7824) (13.0292, 11.1114) (13.1938, 11.4405) (13.3633, 11.7795) knots 0 0 0 0 1 1 1 1
  spline S1306 degree 3 poles (1.8965, 37.7044) (1.732, 37.2108) (1.5674, 36.7173) (1.3979, 36.2087) knots 0 0 0 0 1 1 1 1
  spline S1307 degree 3 poles (1.3979, 36.2087) (0.0817, 36.2087) (-1.2344, 36.2087) (-2.5905, 36.2087) knots 0 0 0 0 1 1 1 1
  spline S1308 degree 3 poles (-2.5905, 36.2087) (-2.755, 36.5378) (-2.9196, 36.8668) (-3.0891, 37.2058) knots 0 0 0 0 1 1 1 1
  spline S1309 degree 3 poles (-3.0891, 37.2058) (-1.4865, 38.0071) (0.1197, 37.733) (1.8965, 37.7044) knots 0 0 0 0 1 1 1 1
  spline S1310 degree 3 poles (-27.0198, -12.1512) (-27.0198, -12.4803) (-27.0198, -12.8093) (-27.0198, -13.1483) knots 0 0 0 0 1 1 1 1
  spline S1311 degree 3 poles (-27.0198, -13.1483) (-28.994, -13.1483) (-30.9683, -13.1483) (-33.0024, -13.1483) knots 0 0 0 0 1 1 1 1
  spline S1312 degree 3 poles (-33.0024, -13.1483) (-32.8379, -12.8193) (-32.6734, -12.4902) (-32.5039, -12.1512) knots 0 0 0 0 1 1 1 1
  spline S1313 degree 3 poles (-32.5039, -12.1512) (-31.5087, -11.9272) (-31.5087, -11.9272) (-30.2915, -11.8085) knots 0 0 0 0 1 1 1 1
  spline S1314 degree 3 poles (-30.2915, -11.8085) (-29.8912, -11.7654) (-29.4908, -11.7223) (-29.0783, -11.678) knots 0 0 0 0 1 1 1 1
  spline S1315 degree 3 poles (-29.0783, -11.678) (-28.0169, -11.6527) (-28.0169, -11.6527) (-27.0198, -12.1512) knots 0 0 0 0 1 1 1 1
  spline S1316 degree 3 poles (-21.0371, 46.6784) (-20.8726, 46.6784) (-20.708, 46.6784) (-20.5385, 46.6784) knots 0 0 0 0 1 1 1 1
  spline S1317 degree 3 poles (-20.5385, 46.6784) (-20.5116, 45.8684) (-20.4923, 45.0582) (-20.4762, 44.2479) knots 0 0 0 0 1 1 1 1
  spline S1318 degree 3 poles (-20.4762, 44.2479) (-20.4647, 43.7968) (-20.4531, 43.3456) (-20.4412, 42.8808) knots 0 0 0 0 1 1 1 1
  spline S1319 degree 3 poles (-20.4412, 42.8808) (-20.5385, 41.6928) (-20.5385, 41.6928) (-21.5356, 40.6957) knots 0 0 0 0 1 1 1 1
  spline S1320 degree 3 poles (-21.5356, 40.6957) (-22.5951, 40.8827) (-22.5951, 40.8827) (-23.5299, 41.1943) knots 0 0 0 0 1 1 1 1
  spline S1321 degree 3 poles (-23.5299, 41.1943) (-23.3037, 41.3588) (-23.0774, 41.5233) (-22.8444, 41.6928) knots 0 0 0 0 1 1 1 1
  spline S1322 degree 3 poles (-22.8444, 41.6928) (-21.6138, 43.2073) (-21.4417, 44.7798) (-21.0371, 46.6784) knots 0 0 0 0 1 1 1 1
  spline S1323 degree 3 poles (36.7954, -12.1512) (36.6309, -12.4803) (36.4664, -12.8093) (36.2968, -13.1483) knots 0 0 0 0 1 1 1 1
  spline S1324 degree 3 poles (36.2968, -13.1483) (35.1576, -13.3548) (35.1576, -13.3548) (33.7729, -13.4599) knots 0 0 0 0 1 1 1 1
  spline S1325 degree 3 poles (33.7729, -13.4599) (33.3147, -13.4972) (32.8565, -13.5345) (32.3844, -13.5729) knots 0 0 0 0 1 1 1 1
  spline S1326 degree 3 poles (32.3844, -13.5729) (32.0302, -13.5973) (31.6761, -13.6217) (31.3113, -13.6469) knots 0 0 0 0 1 1 1 1
  spline S1327 degree 3 poles (31.3113, -13.6469) (31.3113, -13.1533) (31.3113, -12.6597) (31.3113, -12.1512) knots 0 0 0 0 1 1 1 1
  spline S1328 degree 3 poles (31.3113, -12.1512) (33.2965, -11.6257) (34.7922, -11.7319) (36.7954, -12.1512) knots 0 0 0 0 1 1 1 1
  spline S1329 degree 3 poles (7.8792, 4.3011) (8.0437, 4.3011) (8.2082, 4.3011) (8.3777, 4.3011) knots 0 0 0 0 1 1 1 1
  spline S1330 degree 3 poles (8.3777, 4.3011) (8.4047, 3.5847) (8.424, 2.8679) (8.44, 2.1511) knots 0 0 0 0 1 1 1 1
  spline S1331 degree 3 poles (8.44, 2.1511) (8.4516, 1.752) (8.4632, 1.3529) (8.4751, 0.9417) knots 0 0 0 0 1 1 1 1
  spline S1332 degree 3 poles (8.4751, 0.9417) (8.3777, -0.1859) (8.3777, -0.1859) (7.3806, -1.6815) knots 0 0 0 0 1 1 1 1
  spline S1333 degree 3 poles (7.3806, -1.6815) (7.0516, -1.6815) (6.7225, -1.6815) (6.3835, -1.6815) knots 0 0 0 0 1 1 1 1
  spline S1334 degree 3 poles (6.3835, -1.6815) (6.5383, -0.9646) (6.6943, -0.248) (6.8509, 0.4685) knots 0 0 0 0 1 1 1 1
  spline S1335 degree 3 poles (6.8509, 0.4685) (6.9376, 0.8676) (7.0244, 1.2667) (7.1138, 1.6779) knots 0 0 0 0 1 1 1 1
  spline S1336 degree 3 poles (7.1138, 1.6779) (7.3806, 2.8055) (7.3806, 2.8055) (7.8792, 4.3011) knots 0 0 0 0 1 1 1 1
  spline S1337 degree 3 poles (-45.4663, 24.7419) (-44.8082, 24.2484) (-44.1502, 23.7548) (-43.4721, 23.2463) knots 0 0 0 0 1 1 1 1
  spline S1338 degree 3 poles (-43.4721, 23.2463) (-43.6366, 22.5882) (-43.8012, 21.9301) (-43.9707, 21.252) knots 0 0 0 0 1 1 1 1
  spline S1339 degree 3 poles (-43.9707, 21.252) (-44.2997, 21.4166) (-44.6288, 21.5811) (-44.9678, 21.7506) knots 0 0 0 0 1 1 1 1
  spline S1340 degree 3 poles (-44.9678, 21.7506) (-44.9678, 22.0796) (-44.9678, 22.4087) (-44.9678, 22.7477) knots 0 0 0 0 1 1 1 1
  spline S1341 degree 3 poles (-44.9678, 22.7477) (-45.4614, 22.5832) (-45.9549, 22.4187) (-46.4635, 22.2492) knots 0 0 0 0 1 1 1 1
  spline S1342 degree 3 poles (-46.4635, 22.2492) (-46.628, 22.5782) (-46.7925, 22.9072) (-46.962, 23.2463) knots 0 0 0 0 1 1 1 1
  spline S1343 degree 3 poles (-46.962, 23.2463) (-46.633, 23.2463) (-46.3039, 23.2463) (-45.9649, 23.2463) knots 0 0 0 0 1 1 1 1
  spline S1344 degree 3 poles (-45.9649, 23.2463) (-45.8004, 23.7398) (-45.6358, 24.2334) (-45.4663, 24.7419) knots 0 0 0 0 1 1 1 1
  spline S1345 degree 3 poles (-24.0284, 24.2434) (-21.6257, 24.3606) (-19.8092, 23.9701) (-17.5472, 23.2463) knots 0 0 0 0 1 1 1 1
  spline S1346 degree 3 poles (-17.5472, 23.2463) (-17.5472, 23.0817) (-17.5472, 22.9172) (-17.5472, 22.7477) knots 0 0 0 0 1 1 1 1
  spline S1347 degree 3 poles (-17.5472, 22.7477) (-19.357, 22.7477) (-21.1667, 22.7477) (-23.0313, 22.7477) knots 0 0 0 0 1 1 1 1
  spline S1348 degree 3 poles (-23.0313, 22.7477) (-23.0313, 23.0768) (-23.0313, 23.4058) (-23.0313, 23.7448) knots 0 0 0 0 1 1 1 1
  spline S1349 degree 3 poles (-23.0313, 23.7448) (-23.3604, 23.9093) (-23.6894, 24.0739) (-24.0284, 24.2434) knots 0 0 0 0 1 1 1 1
  spline S1350 degree 3 poles (37.7925, -4.1743) (38.1216, -4.6679) (38.4506, -5.1615) (38.7896, -5.67) knots 0 0 0 0 1 1 1 1
  spline S1351 degree 3 poles (38.7896, -5.67) (38.3534, -7.0099) (38.3534, -7.0099) (37.7925, -8.1628) knots 0 0 0 0 1 1 1 1
  spline S1352 degree 3 poles (37.7925, -8.1628) (36.8054, -8.1628) (35.8182, -8.1628) (34.8012, -8.1628) knots 0 0 0 0 1 1 1 1
  spline S1353 degree 3 poles (34.8012, -8.1628) (35.2022, -7.7823) (35.6032, -7.4018) (36.0164, -7.0099) knots 0 0 0 0 1 1 1 1
  spline S1354 degree 3 poles (36.0164, -7.0099) (37.3777, -5.7725) (37.3777, -5.7725) (37.7925, -4.1743) knots 0 0 0 0 1 1 1 1
  spline S1355 degree 3 poles (-64.4115, -5.1714) (-62.1081, -5.5005) (-59.8048, -5.8295) (-57.4317, -6.1685) knots 0 0 0 0 1 1 1 1
  spline S1356 degree 3 poles (-57.4317, -6.1685) (-57.4317, -6.3331) (-57.4317, -6.4976) (-57.4317, -6.6671) knots 0 0 0 0 1 1 1 1
  spline S1357 degree 3 poles (-57.4317, -6.6671) (-60.3931, -6.9139) (-60.3931, -6.9139) (-63.4144, -7.1656) knots 0 0 0 0 1 1 1 1
  spline S1358 degree 3 poles (-63.4144, -7.1656) (-63.4144, -6.8366) (-63.4144, -6.5076) (-63.4144, -6.1685) knots 0 0 0 0 1 1 1 1
  spline S1359 degree 3 poles (-63.4144, -6.1685) (-63.7434, -6.1685) (-64.0724, -6.1685) (-64.4115, -6.1685) knots 0 0 0 0 1 1 1 1
  spline S1360 degree 3 poles (-64.4115, -6.1685) (-64.4115, -5.8395) (-64.4115, -5.5104) (-64.4115, -5.1714) knots 0 0 0 0 1 1 1 1
  spline S1361 degree 3 poles (45.2709, -2.1801) (45.5999, -2.1801) (45.9289, -2.1801) (46.268, -2.1801) knots 0 0 0 0 1 1 1 1
  spline S1362 degree 3 poles (46.268, -2.1801) (45.7744, -4.1544) (45.2808, -6.1287) (44.7723, -8.1628) knots 0 0 0 0 1 1 1 1
  spline S1363 degree 3 poles (44.7723, -8.1628) (44.6078, -8.1628) (44.4433, -8.1628) (44.2737, -8.1628) knots 0 0 0 0 1 1 1 1
  spline S1364 degree 3 poles (44.2737, -8.1628) (44.2467, -7.4463) (44.2274, -6.7295) (44.2114, -6.0127) knots 0 0 0 0 1 1 1 1
  spline S1365 degree 3 poles (44.2114, -6.0127) (44.1999, -5.6136) (44.1883, -5.2145) (44.1764, -4.8034) knots 0 0 0 0 1 1 1 1
  spline S1366 degree 3 poles (44.1764, -4.8034) (44.2737, -3.6758) (44.2737, -3.6758) (45.2709, -2.1801) knots 0 0 0 0 1 1 1 1
  spline S1367 degree 3 poles (-31.5068, 15.2694) (-31.1777, 15.2694) (-30.8487, 15.2694) (-30.5097, 15.2694) knots 0 0 0 0 1 1 1 1
  spline S1368 degree 3 poles (-30.5097, 15.2694) (-30.5097, 13.9399) (-30.5097, 12.6104) (-30.5097, 11.2809) knots 0 0 0 0 1 1 1 1
  spline S1369 degree 3 poles (-30.5097, 11.2809) (-31.0032, 11.2809) (-31.4968, 11.2809) (-32.0053, 11.2809) knots 0 0 0 0 1 1 1 1
  spline S1370 degree 3 poles (-32.0053, 11.2809) (-32.4693, 12.5801) (-32.5783, 13.0967) (-32.0365, 14.3969) knots 0 0 0 0 1 1 1 1
  spline S1371 degree 3 poles (-32.0365, 14.3969) (-31.8617, 14.6848) (-31.6869, 14.9727) (-31.5068, 15.2694) knots 0 0 0 0 1 1 1 1
  spline S1372 degree 3 poles (-55.4375, 16.765) (-55.1084, 16.436) (-54.7794, 16.1069) (-54.4403, 15.7679) knots 0 0 0 0 1 1 1 1
  spline S1373 degree 3 poles (-54.4403, 15.7679) (-54.6163, 14.0521) (-54.9617, 13.2409) (-55.936, 11.7795) knots 0 0 0 0 1 1 1 1
  spline S1374 degree 3 poles (-55.936, 11.7795) (-56.2651, 11.7795) (-56.5941, 11.7795) (-56.9331, 11.7795) knots 0 0 0 0 1 1 1 1
  spline S1375 degree 3 poles (-56.9331, 11.7795) (-57.0976, 12.273) (-57.2622, 12.7666) (-57.4317, 13.2751) knots 0 0 0 0 1 1 1 1
  spline S1376 degree 3 poles (-57.4317, 13.2751) (-56.9381, 13.2751) (-56.4445, 13.2751) (-55.936, 13.2751) knots 0 0 0 0 1 1 1 1
  spline S1377 degree 3 poles (-55.936, 13.2751) (-55.7715, 14.4268) (-55.607, 15.5785) (-55.4375, 16.765) knots 0 0 0 0 1 1 1 1
  spline S1378 degree 3 poles (-64.91, 24.7419) (-64.581, 24.5774) (-64.2519, 24.4129) (-63.9129, 24.2434) knots 0 0 0 0 1 1 1 1
  spline S1379 degree 3 poles (-63.9129, 24.2434) (-64.9001, 22.7627) (-64.9001, 22.7627) (-65.9071, 21.252) knots 0 0 0 0 1 1 1 1
  spline S1380 degree 3 poles (-65.9071, 21.252) (-66.5652, 21.5811) (-67.2233, 21.9101) (-67.9014, 22.2492) knots 0 0 0 0 1 1 1 1
  spline S1381 degree 3 poles (-67.9014, 22.2492) (-66.9142, 23.0718) (-65.9271, 23.8944) (-64.91, 24.7419) knots 0 0 0 0 1 1 1 1
  spline S1382 degree 3 poles (-11.066, 27.2347) (-10.5724, 27.0702) (-10.0788, 26.9057) (-9.5703, 26.7362) knots 0 0 0 0 1 1 1 1
  spline S1383 degree 3 poles (-9.5703, 26.7362) (-10.2627, 25.0629) (-11.0245, 24.207) (-12.5616, 23.2463) knots 0 0 0 0 1 1 1 1
  spline S1384 degree 3 poles (-12.5616, 23.2463) (-12.8907, 23.2463) (-13.2197, 23.2463) (-13.5588, 23.2463) knots 0 0 0 0 1 1 1 1
  spline S1385 degree 3 poles (-13.5588, 23.2463) (-13.5588, 23.5753) (-13.5588, 23.9044) (-13.5588, 24.2434) knots 0 0 0 0 1 1 1 1
  spline S1386 degree 3 poles (-13.5588, 24.2434) (-13.0652, 24.5724) (-12.5716, 24.9015) (-12.0631, 25.2405) knots 0 0 0 0 1 1 1 1
  spline S1387 degree 3 poles (-12.0631, 25.2405) (-11.4686, 26.2626) (-11.4686, 26.2626) (-11.066, 27.2347) knots 0 0 0 0 1 1 1 1
  spline S1388 degree 3 poles (-21.5356, 34.2145) (-21.7002, 33.5564) (-21.8647, 32.8983) (-22.0342, 32.2203) knots 0 0 0 0 1 1 1 1
  spline S1389 degree 3 poles (-22.0342, 32.2203) (-22.1987, 32.7138) (-22.3633, 33.2074) (-22.5328, 33.7159) knots 0 0 0 0 1 1 1 1
  spline S1390 degree 3 poles (-22.5328, 33.7159) (-23.1035, 33.4537) (-23.1035, 33.4537) (-23.6857, 33.1862) knots 0 0 0 0 1 1 1 1
  spline S1391 degree 3 poles (-23.6857, 33.1862) (-25.0255, 32.7188) (-25.0255, 32.7188) (-26.5212, 33.2174) knots 0 0 0 0 1 1 1 1
  spline S1392 degree 3 poles (-26.5212, 33.2174) (-24.6641, 34.5439) (-23.7399, 34.9073) (-21.5356, 34.2145) knots 0 0 0 0 1 1 1 1
  spline S1393 degree 3 poles (-52.9447, -8.6613) (-52.7802, -8.9904) (-52.6156, -9.3194) (-52.4461, -9.6584) knots 0 0 0 0 1 1 1 1